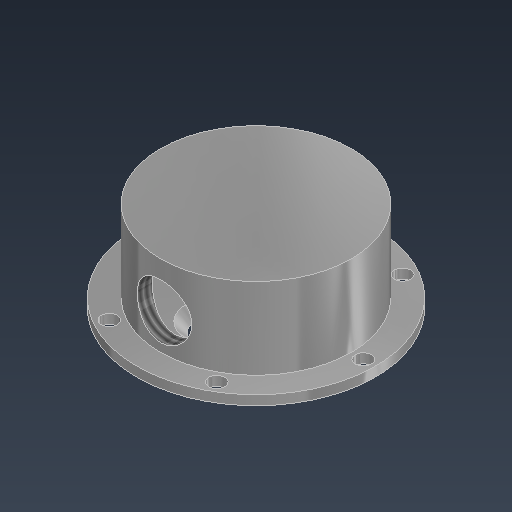
# Autodesk Inventor part: P011-Chapeau_chambre
Saved by Autodesk Inventor 2021.3 (Build 253353000, 353)
## iProperties
Created: 2022-03-24
Part Number: P011-Chapeau_chambre
Material: Aluminium
Document SubType Name: Modeling
Designer: Maintenant Prêt
Density: 2.7 g/cm^3
Appearance: Aluminum - Dark
Author: Maintenant Prêt
Autodesk Inventor part; units mm, degrees
ref_plane "YZ Plane" through (0, 0, 0) normal (1, 0, 0) x (0, 1, 0)
ref_plane "XY Plane" through (0, 0, 0) normal (0, 0, 1) x (1, 0, 0)
sketch "Sketch6" plane through (0, 0, 0) normal (1, 0, 0) x (0, 1, 0)
  line L0 (0, 0) -> (25, 0)
  line L1 (25, 0) -> (25, 2)
  line L2 (25, 2) -> (20, 2)
  line L3 (20, 2) -> (20, 19)
  line L4 (20, 19) -> (0, 19)
  line L5 (0, 19) -> (0, 17)
  line L6 (0, 17) -> (17, 17)
  line L7 (17, 17) -> (17, 2)
  line L8 (17, 2) -> (0, 2)
  line L9 (0, 0) -> (0, 2)
  line L10 (17, 2) -> (20, 2) construction
  line L11 (0, -3.8) -> (0, 22.8) construction
  dimension "d11" = 2
  dimension "d13" = 34
  dimension "d15" = 15
  dimension "d16" = 5
  dimension "d28" = 3
  constraints: 22 end point, 8 perpendicular, 3 point on line, 2 horizontal, 1 parallel
  measures "d11" distance of L0.end L1.end
  measures "d13" diameter of L7 L11
  measures "d15" distance of L6.end L7.end
  measures "d16" distance of L1.end L2.end
  measures "d28" distance of L7.end L2.end
revolve "Revolution1" add sketch "Sketch6" angle 360 about axis through (0, 0, -10) along (0, 0, 1)
ref_plane "Work Plane1" through (0, 20, 0) normal (0, 1, 0) x (-1, 0, 0)
sketch "Sketch8" plane through (0, 20, 0) normal (0, 1, 0) x (-1, 0, 0)
  line L0 (-17, 2) -> (17, 2) construction
  line L1 (-17, 17) -> (17, 17) construction
  line L2 (-17, 17) -> (17, 2) construction
  line L3 (-17, 2) -> (17, 17) construction
  point P0 (0, 0)
  point P1 (0, 9.5)
  constraints: 4 end point, 2 midpoint
hole "Hole1" at (0, 20, 9.5) direction (0, -1, 0) diameter 11.445 end through all thread size "G 1/4-19" standard "BSP Pipe Threads"
sketch "Sketch9" plane through (0, 0, 0) normal (0, 1, 0) x (-1, 0, 0)
  line L0 (-17, 2) -> (17, 2) construction
  line L1 (-17, 17) -> (17, 17) construction
  line L2 (-17, 17) -> (17, 17)
  line L3 (17, 17) -> (17, 2)
  line L4 (17, 2) -> (-17, 2)
  line L5 (-17, 2) -> (-17, 17)
  point P0 (0, 0)
  constraints: 8 end point, 2 parallel, 1 horizontal, 1 perpendicular, 2 other
extrude "Extrusion5" add sketch "Sketch9" along normal mid plane 1
sketch "Sketch10" plane through (0, 0, 0) normal (0, 0, -1) x (-1, 0, 0)
  line L0 (16.9926, 0.5) -> (-16.9926, 0.5) construction
  arc A0 (16.9926, 0.5) -> (-16.9926, 0.5) centre (0, 0) ccw construction
  line L1 (-16.9926, -0.5) -> (16.9926, -0.5) construction
  arc A1 (-16.9926, -0.5) -> (16.9926, -0.5) centre (0, 0) ccw construction
  line L2 (0, 17) -> (0, 8.75) construction
  line L3 (0, 8.75) -> (0, 0.5) construction
  line L4 (0, -0.5) -> (0, -8.75) construction
  line L5 (0, -8.75) -> (0, -17) construction
  constraints: 8 end point, 4 collinear, 2 coincident, 2 midpoint, 2 point on circle
hole "Hole2" at (0, 8.75, 0) at (0, -8.75, 0) direction (0, 0, 1) diameter 8 depth 2
chamfer "Chamfer1" distance 2 angle 45 2 edges at (0, 4.75, 0) (0, -12.75, 2)
sketch "Sketch11" plane through (0, 0, 2) normal (0, 0, 1) x (1, 0, 0)
  circle A0 centre (0, 0) radius 20 construction
  circle A1 centre (0, 0) radius 25 construction
  circle A2 centre (0, 0) radius 22.5 construction
  line L0 (-35, 0) -> (35, 0) construction
  point P0 (22.5, 0)
  point P1 (11.25, 19.4856)
  point P2 (-11.25, 19.4856)
  point P3 (-22.5, 0)
  point P4 (-11.25, -19.4856)
  point P5 (11.25, -19.4856)
  dimension "d43" = 45
  dimension "d41" = 40
  dimension "d42" = 50
  dimension "d46" = 360
  constraints: 1 coincident, 1 horizontal alignment, 1 point on line, 9 other
  measures "d41" diameter of A0
  measures "d42" diameter of A1
hole "Hole3" at (22.5, 0, 2) at (11.25, 19.4856, 2) at (-11.25, 19.4856, 2) at (-22.5, 0, 2) at (-11.25, -19.4856, 2) at (11.25, -19.4856, 2) direction (0, 0, -1) diameter 3.4 depth 2 clearance for "Flat Head Machine Screw" size "M3" standard "Ansi Metric M Profile"
equation "\"d28\" = 1.5 * d11"
equation "\"d43\" = 0.5 * d42 + 0.5 * d41"
body "Solid2"
